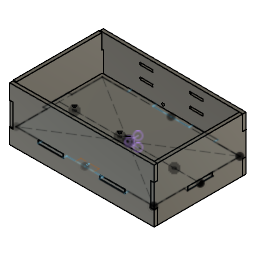
Backing Plate and Box (Autodesk Fusion 360 design; units mm, degrees)
part number: 2026-02-17-21-20-32-268
Autodesk Fusion 360 part; units mm, degrees
sketch "Base Plate" plane through (0, 0, 0) normal (0, 0, 1) x (1, 0, 0)
  line L0 (136.5, 85.5) -> (-136.5, 85.5) construction
  line L1 (-136.5, 85.5) -> (-136.5, -85.5) construction
  line L2 (-136.5, -85.5) -> (136.5, -85.5) construction
  line L3 (136.5, -85.5) -> (136.5, 85.5) construction
  line L4 (136.5, 85.5) -> (-136.5, -85.5) construction
  line L5 (-136.5, 85.5) -> (136.5, -85.5) construction
  line L6 (-35.8624, -85.7255) -> (-35.8624, -92.1)
  line L7 (-35.8624, -92.1) -> (-85.8619, -92.1)
  line L8 (-85.8619, -92.1) -> (-85.8619, -85.5)
  line L9 (-136.5, -85.5) -> (-85.8619, -85.5)
  line L10 (-35.8624, -85.7255) -> (0, -85.5)
  line L11 (0, 2.5) -> (0, 20)
  line L12 (136.5, -85.5) -> (85.8619, -85.5)
  line L13 (85.8619, -92.1) -> (85.8619, -85.5)
  line L14 (35.8624, -92.1) -> (85.8619, -92.1)
  line L15 (35.8624, -85.7255) -> (35.8624, -92.1)
  line L16 (35.8624, -85.7255) -> (0, -85.5)
  line L17 (20, 0) -> (2.5, 0)
  line L18 (-35.8624, 85.7255) -> (-35.8624, 92.1)
  line L19 (35.8624, 85.7255) -> (0, 85.5)
  line L20 (-136.5, 85.5) -> (136.5, 85.5) construction
  line L21 (-35.8624, 92.1) -> (-85.8619, 92.1)
  line L22 (35.8624, 92.1) -> (85.8619, 92.1)
  line L23 (136.5, 85.5) -> (85.8619, 85.5)
  line L24 (-136.5, 85.5) -> (-85.8619, 85.5)
  line L25 (35.8624, 85.7255) -> (35.8624, 92.1)
  line L26 (-35.8624, 85.7255) -> (0, 85.5)
  line L27 (-85.8619, 92.1) -> (-85.8619, 85.5)
  line L28 (85.8619, 92.1) -> (85.8619, 85.5)
  line L29 (-136.5, 25) -> (-143.1, 25)
  line L30 (-143.1, 25) -> (-143.1, 0)
  line L31 (-136.5, 25) -> (-136.5, 85.5)
  line L32 (-136.5, -25) -> (-136.5, -85.5)
  line L33 (-143.1, -25) -> (-143.1, 0)
  line L34 (-136.5, -25) -> (-143.1, -25)
  line L35 (136.5, -25) -> (143.1, -25)
  line L36 (143.1, -25) -> (143.1, 0)
  line L37 (136.5, 25) -> (136.5, 85.5)
  line L38 (136.5, -25) -> (136.5, -85.5)
  line L39 (143.1, 25) -> (143.1, 0)
  line L40 (136.5, 85.5) -> (136.5, -85.5) construction
  line L41 (136.5, 25) -> (143.1, 25)
  line L42 (-136.5, -85.5) -> (-136.5, 0.3) construction
  line L43 (-136.5, 0.3) -> (136.5, 0.3) construction
  line L44 (-136.5, 0.3) -> (-106.5, 0.3) construction
  line L45 (-106.5, 0.3) -> (-16.5, 0.3) construction
  line L46 (-16.5, 0.3) -> (91.5, 0.3) construction
  line L47 (91.5, 0.3) -> (136.5, 0.3) construction
  circle A0 centre (-106.5, 0.3) radius 2.45
  circle A1 centre (-16.5, 0.3) radius 2.45
  circle A2 centre (91.5, 0.3) radius 2.45
  line L48 (-17.9312, -85.6127) -> (17.9312, -85.6127) construction
  line L49 (17.9312, -85.6127) -> (17.9312, -75.542) construction
  line L50 (17.9312, -75.542) -> (-17.9312, -75.542) construction
  line L51 (-17.9312, -75.542) -> (-17.9312, -85.6127) construction
  point P0 (-136.5, -85.5)
  point P1 (136.5, -85.5)
  dimension "d1" = 273
  dimension "d2" = 171
  dimension "d3" = 50
  dimension "d4" = 6.6
  dimension "d6" = 6.6
  dimension "d7" = 25
  dimension "d8" = 85.8
  dimension "d9" = 273
  dimension "d10" = 30
  dimension "d11" = 90
  dimension "d12" = 108
  dimension "d13" = 45
  dimension "d16" = 4.9
  dimension "d17" = 4.9
  dimension "d18" = 4.9
  dimension "d23" = 7
  text T0 "B" font "Arial" height 7 align centre top in box 35.8624 x 10.0707 at (-17.9312, -85.6127) x (1, 0) y (0, 1) spacing 1 kerned
  constraint horizontal L0
  constraint perpendicular L0 L1
  constraint parallel L0 L2
  constraint parallel L1 L3
  constraint coincident L4 origin
  constraint coincident L5 origin
  constraint vertical L6
  constraint horizontal L7
  constraint vertical L8
  constraint coincident L2 L8.end
  constraint midpoint L2 L10.end
  constraint symmetric P0 L11 P1
  constraint symmetric L8.end L11 L12.end
  constraint symmetric L6.start L11 L15.start
  constraint symmetric L6.end L11 L14.start
  constraint symmetric L7.end L11 L13.start
  constraint symmetric L10.end L11 L16.end
  constraint symmetric P0 L17 L0.end
  constraint symmetric P1 L17 L0.start
  constraint symmetric L8.end L17 L24.end
  constraint symmetric L6.start L17 L18.start
  constraint symmetric L6.end L17 L18.end
  constraint symmetric L7.end L17 L21.end
  constraint symmetric L10.end L17 L19.end
  constraint symmetric L12.end L17 L23.end
  constraint symmetric L13.start L17 L22.end
  constraint symmetric L14.start L17 L22.start
  constraint symmetric L15.start L17 L19.start
  constraint perpendicular L29 L30
  constraint symmetric L0.end L17 P0
  constraint symmetric L17 L0.end P0
  constraint symmetric L17 L29.start L32.start
  constraint symmetric L17 L29.end L33.start
  constraint symmetric L17 L30.end L33.end
  constraint symmetric L0.end L11 L0.start
  constraint symmetric L11 L0.end L0.start
  constraint symmetric L11 L29.start L37.start
  constraint symmetric L11 L29.end L39.start
  constraint symmetric L11 L30.end L36.end
  constraint symmetric L11 P0 P1
  constraint symmetric L11 L32.start L35.start
  constraint symmetric L11 L33.start L35.end
  constraint parallel L1 L42
  constraint horizontal L43
  constraint horizontal L44
  constraint perpendicular L1 L45
  constraint horizontal L46
  constraint perpendicular L29 L31
  constraint coincident L30.end L33.end
  constraint perpendicular L0 L31
  constraint coincident L44.end L45.start
  constraint coincident L45.end L46.start
  constraint coincident L46.end L47.start
  constraint midpoint L16
  constraint midpoint L10
  measures "d1" distance of P0 P1
  measures "d2" distance of L0.end P0
  measures "d3" distance of L8.end L6.start
  measures "d4" distance of L8.end L7.end
  measures "d6" distance of L29.start L29.end
  measures "d7" distance of L29.end L30.end
  measures "d8" distance of P0 L42.end
  measures "d9" distance of L42.end L43.end
  measures "d10" distance of L42.end L44.end
  measures "d11" distance of L44.end L45.end
  measures "d12" distance of L45.end L46.end
  measures "d13" distance of L43.end L46.end
  measures "d16" diameter of A0
  measures "d17" diameter of A1
  measures "d18" diameter of A2
extrude "Extrude1" add sketch "Base Plate" along normal blind 6.6 makes body 1
fillet "Fillet1" radius 1 16 edges at (-85.8619, -92.1, 3.3) (-35.8624, -92.1, 3.3) (35.8624, -92.1, 3.3) (85.8619, -92.1, 3.3) (136.5, -85.5, 3.3) (-136.5, -85.5, 3.3) (-143.1, -25, 3.3) (-143.1, 25, 3.3) (-136.5, 85.5, 3.3) (-85.8619, 92.1, 3.3) (-35.8624, 92.1, 3.3) (35.8624, 92.1, 3.3) (85.8619, 92.1, 3.3) (136.5, 85.5, 3.3) (143.1, 25, 3.3) (143.1, -25, 3.3) on bodies 1
extrude "Extrude2" cut sketch "Base Plate" along normal blind 6.6 text T0 bodies 1 makes body 2 at (-1.7166, -77.0732, 2.2) makes body 3 at (36.9029, -29.1248, 0)
sketch "For Cutting" plane through (0, 0, 6.6) normal (0, 0, 1) x (-1, 0, 0)
  line L0 (2.6429, 82.542) -> (2.6429, 75.542)
  line L1 (2.6429, 75.542) -> (0.0167, 75.542)
  spline S0 degree 3 poles (0.0167, 75.542) (-0.2266, 75.5465) (-0.6666, 75.5545) (-1.0836, 75.6927) (-1.2701, 75.7545) knots 0 0 0 0 0.072475 0.131086 0.131086 0.131086 0.131086
  spline S1 degree 3 poles (-1.2701, 75.7545) (-1.4227, 75.8345) (-1.7265, 75.9939) (-1.9287, 76.2708) (-2.0293, 76.4087) knots 0 0 0 0 0.050943 0.101413 0.101413 0.101413 0.101413
  spline S2 degree 3 poles (-2.0293, 76.4087) (-2.1094, 76.5559) (-2.2664, 76.8446) (-2.2916, 77.1721) (-2.3039, 77.3326) knots 0 0 0 0 0.049654 0.097362 0.097362 0.097362 0.097362
  spline S3 degree 3 poles (-2.3039, 77.3326) (-2.2934, 77.4806) (-2.2721, 77.7795) (-2.1314, 78.0442) (-2.0604, 78.1778) knots 0 0 0 0 0.043994 0.088828 0.088828 0.088828 0.088828
  spline S4 degree 3 poles (-2.0604, 78.1778) (-1.9655, 78.3051) (-1.7672, 78.5714) (-1.4766, 78.7332) (-1.325, 78.8176) knots 0 0 0 0 0.047078 0.098463 0.098463 0.098463 0.098463
  spline S5 degree 3 poles (-1.325, 78.8176) (-1.5218, 78.8871) (-1.899, 79.0205) (-2.1712, 79.3128) (-2.3015, 79.4527) knots 0 0 0 0 0.061554 0.118026 0.118026 0.118026 0.118026
  spline S6 degree 3 poles (-2.3015, 79.4527) (-2.4011, 79.6112) (-2.6046, 79.9352) (-2.63, 80.3174) (-2.6429, 80.5127) knots 0 0 0 0 0.055236 0.112931 0.112931 0.112931 0.112931
  spline S7 degree 3 poles (-2.6429, 80.5127) (-2.6346, 80.6729) (-2.6183, 80.9898) (-2.4958, 81.2824) (-2.4352, 81.4271) knots 0 0 0 0 0.047734 0.094399 0.094399 0.094399 0.094399
  spline S8 degree 3 poles (-2.4352, 81.4271) (-2.3649, 81.5575) (-2.2317, 81.805) (-2.0213, 81.9909) (-1.9219, 82.0789) knots 0 0 0 0 0.044041 0.083545 0.083545 0.083545 0.083545
  spline S9 degree 3 poles (-1.9219, 82.0789) (-1.8097, 82.1515) (-1.5719, 82.3055) (-1.2994, 82.3837) (-1.1555, 82.425) knots 0 0 0 0 0.039883 0.084504 0.084504 0.084504 0.084504
  spline S10 degree 3 poles (-1.1555, 82.425) (-0.9851, 82.4591) (-0.6126, 82.5336) (-0.2325, 82.539) (-0.0263, 82.542) knots 0 0 0 0 0.052016 0.113741 0.113741 0.113741 0.113741
  line L2 (-0.0263, 82.542) -> (2.6429, 82.542)
  arc A0 (-142.1, 25) -> (-143.1, 24) centre (-142.1, 24) ccw
  line L3 (-143.1, 24) -> (-143.1, -24)
  arc A1 (-143.1, -24) -> (-142.1, -25) centre (-142.1, -24) ccw
  line L4 (-142.1, -25) -> (-136.5, -25)
  line L5 (-136.5, -25) -> (-136.5, -84.5)
  arc A2 (-136.5, -84.5) -> (-135.5, -85.5) centre (-135.5, -84.5) ccw
  line L6 (-135.5, -85.5) -> (-85.8619, -85.5)
  line L7 (-85.8619, -85.5) -> (-85.8619, -91.1)
  arc A3 (-85.8619, -91.1) -> (-84.8619, -92.1) centre (-84.8619, -91.1) ccw
  line L8 (-84.8619, -92.1) -> (-36.8624, -92.1)
  arc A4 (-36.8624, -92.1) -> (-35.8624, -91.1) centre (-36.8624, -91.1) ccw
  line L9 (-35.8624, -91.1) -> (-35.8624, -85.7255)
  line L10 (-35.8624, -85.7255) -> (0, -85.5)
  line L11 (0, -85.5) -> (35.8624, -85.7255)
  line L12 (35.8624, -85.7255) -> (35.8624, -91.1)
  arc A5 (35.8624, -91.1) -> (36.8624, -92.1) centre (36.8624, -91.1) ccw
  line L13 (36.8624, -92.1) -> (84.8619, -92.1)
  arc A6 (84.8619, -92.1) -> (85.8619, -91.1) centre (84.8619, -91.1) ccw
  line L14 (85.8619, -91.1) -> (85.8619, -85.5)
  line L15 (85.8619, -85.5) -> (135.5, -85.5)
  arc A7 (135.5, -85.5) -> (136.5, -84.5) centre (135.5, -84.5) ccw
  line L16 (136.5, -84.5) -> (136.5, -25)
  line L17 (136.5, -25) -> (142.1, -25)
  arc A8 (142.1, -25) -> (143.1, -24) centre (142.1, -24) ccw
  line L18 (143.1, -24) -> (143.1, 24)
  arc A9 (143.1, 24) -> (142.1, 25) centre (142.1, 24) ccw
  line L19 (142.1, 25) -> (136.5, 25)
  line L20 (136.5, 25) -> (136.5, 84.5)
  arc A10 (136.5, 84.5) -> (135.5, 85.5) centre (135.5, 84.5) ccw
  line L21 (135.5, 85.5) -> (85.8619, 85.5)
  line L22 (85.8619, 85.5) -> (85.8619, 91.1)
  arc A11 (85.8619, 91.1) -> (84.8619, 92.1) centre (84.8619, 91.1) ccw
  line L23 (84.8619, 92.1) -> (36.8624, 92.1)
  arc A12 (36.8624, 92.1) -> (35.8624, 91.1) centre (36.8624, 91.1) ccw
  line L24 (35.8624, 91.1) -> (35.8624, 85.7255)
  line L25 (35.8624, 85.7255) -> (0, 85.5)
  line L26 (0, 85.5) -> (-35.8624, 85.7255)
  line L27 (-35.8624, 85.7255) -> (-35.8624, 91.1)
  arc A13 (-35.8624, 91.1) -> (-36.8624, 92.1) centre (-36.8624, 91.1) ccw
  line L28 (-36.8624, 92.1) -> (-84.8619, 92.1)
  arc A14 (-84.8619, 92.1) -> (-85.8619, 91.1) centre (-84.8619, 91.1) ccw
  line L29 (-85.8619, 91.1) -> (-85.8619, 85.5)
  line L30 (-85.8619, 85.5) -> (-135.5, 85.5)
  arc A15 (-135.5, 85.5) -> (-136.5, 84.5) centre (-135.5, 84.5) ccw
  line L31 (-136.5, 84.5) -> (-136.5, 25)
  line L32 (-136.5, 25) -> (-142.1, 25)
  circle A16 centre (106.5, -0.3) radius 2.45
  circle A17 centre (16.5, -0.3) radius 2.45
  circle A18 centre (-91.5, -0.3) radius 2.45
sketch "Top/Bottom Plate" plane through (0.5375, 85.4966, 0) normal (0.006286, 0.99998, 0) x (-0.99998, 0.006286, 0)
  line L0 (36.4006, 0) -> (36.4006, 6.6)
  line L1 (36.4344, 6.6) -> (36.4344, 0)
  line L2 (86.4329, 0) -> (86.4329, 6.6)
  line L3 (-85.2875, 6.6) -> (-85.2875, 0)
  line L4 (-35.289, 0) -> (-35.289, 6.6)
  line L5 (37.4407, 6.6) -> (85.4392, 6.6)
  line L6 (36.4407, 0) -> (86.4392, 0)
  line L7 (-35.2827, 0) -> (-85.2812, 0)
  line L8 (-84.2813, 6.6) -> (-36.2827, 6.6)
  line L9 (-135.9661, 6.6) -> (-135.9661, 0)
  line L10 (137.0285, 0) -> (137.0285, 6.6)
  line L11 (-85.2875, 6.6) -> (-35.289, 6.6)
  line L12 (-35.289, 6.6) -> (-35.289, 0)
  line L13 (-35.289, 0) -> (-85.2875, 0)
  line L14 (-85.2875, 0) -> (-85.2875, 6.6)
  line L15 (36.4344, 6.6) -> (86.4329, 6.6)
  line L16 (86.4329, 6.6) -> (86.4329, 0)
  line L17 (86.4329, 0) -> (36.4344, 0)
  line L18 (-135.9661, 6.6) -> (-135.9661, 76.6) construction
  line L19 (-135.9661, 0) -> (-135.9661, -30) construction
  line L20 (137.0285, 6.6) -> (137.0285, 76.6) construction
  line L21 (137.0285, 0) -> (137.0285, -30) construction
  line L22 (-135.9661, 76.6) -> (137.0285, 76.6)
  line L23 (137.0285, 76.6) -> (137.0285, -30) construction
  line L24 (137.0285, -30) -> (-135.9661, -30)
  line L25 (-135.9661, -30) -> (-135.9661, 76.6) construction
  line L26 (-135.9661, 76.6) -> (-142.5661, 76.6)
  line L27 (-142.5661, 76.6) -> (-142.5661, 46.6)
  line L28 (-142.5661, 46.6) -> (-135.9661, 46.6)
  line L29 (-135.9661, -30) -> (-142.5661, -30)
  line L30 (-142.5661, -30) -> (-142.5661, 0)
  line L31 (-142.5661, 0) -> (-135.9661, 0)
  line L32 (-135.9661, 0) -> (-135.9661, 46.6)
  line L33 (0, 1.75) -> (0, 22.5)
  line L34 (135.9661, 76.6) -> (142.5661, 76.6)
  line L35 (142.5661, 76.6) -> (142.5661, 46.6)
  line L36 (142.5661, 46.6) -> (135.9661, 46.6)
  line L37 (135.9661, 0) -> (135.9661, 46.6)
  line L38 (142.5661, 0) -> (135.9661, 0)
  line L39 (142.5661, -30) -> (142.5661, 0)
  line L40 (135.9661, -30) -> (142.5661, -30)
  dimension "d27" = 70
  dimension "d28" = 30
  dimension "d29" = 70
  dimension "d30" = 30
  dimension "d33" = 6.6
  dimension "d34" = 30
  dimension "d35" = 6.6
  dimension "d36" = 30
  constraint horizontal L11
  constraint vertical L12
  constraint horizontal L13
  constraint vertical L14
  constraint coincident L4.start L12.end
  constraint coincident L3.start L11.start
  constraint horizontal L15
  constraint vertical L16
  constraint horizontal L17
  constraint coincident L2.start L16.end
  constraint coincident L1.start L15.start
  constraint vertical L18
  constraint coincident L9.start L18.start
  constraint coincident L9.end L19.start
  constraint parallel L9 L19
  constraint coincident L10.end L20.start
  constraint parallel L10 L20
  constraint coincident L10.start L21.start
  constraint parallel L10 L21
  constraint horizontal L22
  constraint vertical L23
  constraint horizontal L24
  constraint vertical L25
  constraint horizontal L26
  constraint vertical L27
  constraint horizontal L28
  constraint horizontal L29
  constraint vertical L30
  constraint horizontal L31
  constraint symmetric L18.end L33 L34.start
  constraint symmetric L9.end L33 L37.start
  constraint symmetric L19.end L33 L40.start
  constraint symmetric L26.end L33 L34.end
  constraint symmetric L27.end L33 L35.end
  constraint symmetric L28.end L33 L36.end
  constraint symmetric L29.end L33 L39.start
  constraint symmetric L30.end L33 L38.start
  measures "d27" distance of L9.start L18.end
  measures "d28" distance of L9.end L19.end
  measures "d29" distance of L10.end L20.end
  measures "d30" distance of L10.start L21.end
  measures "d33" distance of L18.end L26.end
  measures "d34" distance of L18.end L28.end
  measures "d35" distance of L19.end L29.end
  measures "d36" distance of L19.end L9.end
extrude "Extrude5" add sketch "Top/Bottom Plate" along normal blind 6.6 separate body makes body 4
mirror "Mirror2" about plane through (0, 0, 0) normal (0, 1, 0) of bodies 4 makes body 5
sketch "Left/Right Plate" plane through (136.5, 0, 0) normal (1, 0, 0) x (0, 1, 0)
  line L0 (25, 0) -> (25, 6.6)
  line L1 (-25, 6.6) -> (-25, 0)
  line L2 (-84.6004, 0) -> (-91.2002, 0)
  line L3 (-84.6004, 46.6) -> (-91.2002, 46.6)
  line L4 (84.6004, 46.6) -> (91.2002, 46.6)
  line L5 (84.6004, 0) -> (91.2002, 0)
  line L6 (-84.6004, 76.6) -> (84.6004, 76.6)
  line L7 (84.6004, 76.6) -> (84.6004, -30) construction
  line L8 (84.6004, -30) -> (-84.6004, -30)
  line L9 (-84.6004, -30) -> (-84.6004, 76.6) construction
  line L10 (-91.2002, 46.6) -> (-84.6004, 46.6)
  line L11 (-84.6004, 0) -> (-91.2002, 0)
  line L12 (-91.2002, 0) -> (-91.2002, 46.6)
  line L13 (84.6004, 46.6) -> (91.2002, 46.6)
  line L14 (91.2002, 46.6) -> (91.2002, 0)
  line L15 (91.2002, 0) -> (84.6004, 0)
  line L16 (-84.6004, 46.6) -> (-84.6004, 76.6)
  line L17 (-84.6004, 0) -> (-84.6004, -30)
  line L18 (84.6004, 0) -> (84.6004, -30)
  line L19 (84.6004, 46.6) -> (84.6004, 76.6)
  line L20 (-25, 6.6) -> (25, 6.6)
  line L21 (25, 6.6) -> (25, 0)
  line L22 (25, 0) -> (-25, 0)
  line L23 (-25, 0) -> (-25, 6.6)
  point P0 (-84.6004, 76.6)
  point P1 (-84.6004, -30)
  point P2 (84.6004, -30)
  point P3 (84.6004, 76.6)
  point P4 (-84.6004, 46.6)
  point P5 (-91.2002, 0)
  point P6 (91.2002, 0)
  point P7 (84.6419, 46.6)
  constraint horizontal L6
  constraint vertical L7
  constraint horizontal L8
  constraint vertical L9
  constraint coincident P2 L7.end
  constraint coincident P0 L6.start
  constraint horizontal L10
  constraint horizontal L11
  constraint vertical L12
  constraint coincident L2.start L11.start
  constraint coincident L3.end L10.start
  constraint horizontal L13
  constraint vertical L14
  constraint horizontal L15
  constraint coincident P6 L5.end
  constraint coincident L4.start L13.start
  constraint coincident P4 L3.start
  constraint coincident P1 L8.end
  constraint coincident L5.start L15.end
  constraint coincident P3 L6.end
  constraint horizontal L20
  constraint vertical L21
  constraint horizontal L22
  constraint vertical L23
  constraint coincident L0.start L21.end
  constraint coincident L1.start L20.start
extrude "Extrude6" add sketch "Left/Right Plate" along normal blind 6.6 separate body makes body 6
mirror "Mirror3" about plane through (0, 0, 0) normal (1, 0, 0) of bodies 6 makes body 7
sketch "Top Plate Detail" plane through (0.579, 92.0965, 0) normal (0.006286, 0.99998, 0) x (-0.99998, 0.006286, 0)
  line L0 (36.4344, 0) -> (36.4344, 6.6)
  line L1 (36.4344, 6.6) -> (86.4329, 6.6)
  line L2 (86.4329, 6.6) -> (86.4329, 0)
  line L3 (86.4329, 0) -> (36.4344, 0)
  line L4 (-35.289, 0) -> (-85.2875, 0)
  line L5 (-85.2875, 0) -> (-85.2875, 6.6)
  line L6 (-85.2875, 6.6) -> (-35.289, 6.6)
  line L7 (-35.289, 6.6) -> (-35.289, 0)
  line L8 (-142.5661, -30) -> (142.5661, -30)
  line L9 (142.5661, -30) -> (142.5661, 0)
  line L10 (142.5661, 0) -> (135.9661, 0)
  line L11 (135.9661, 0) -> (135.9661, 46.6)
  line L12 (135.9661, 46.6) -> (142.5661, 46.6)
  line L13 (142.5661, 46.6) -> (142.5661, 76.6)
  line L14 (142.5661, 76.6) -> (-142.5661, 76.6)
  line L15 (-142.5661, 76.6) -> (-142.5661, 46.6)
  line L16 (-142.5661, 46.6) -> (-135.9661, 46.6)
  line L17 (-135.9661, 46.6) -> (-135.9661, 0)
  line L18 (-135.9661, 0) -> (-142.5661, 0)
  line L19 (-142.5661, 0) -> (-142.5661, -30)
  line L20 (0, -30) -> (0, 76.6) construction
  line L21 (-91.4963, 0) -> (-91.4963, 13) construction
  line L22 (16.5016, 0) -> (16.5016, 13) construction
  circle A0 centre (-91.4963, 13) radius 2.6
  circle A1 centre (16.5016, 13) radius 2.6
  line L23 (0, 0) -> (-50, 0) construction
  line L24 (-50, 0) -> (-50, -15) construction
  line L25 (-37, -12.9) -> (-63, -12.9)
  line L26 (-63, -12.9) -> (-63, -17.1)
  line L27 (-63, -17.1) -> (-37, -17.1)
  line L28 (-37, -17.1) -> (-37, -12.9)
  line L29 (-37, -12.9) -> (-63, -17.1) construction
  line L30 (-63, -12.9) -> (-37, -17.1) construction
  line L31 (37, -12.9) -> (63, -12.9)
  line L32 (37, -17.1) -> (37, -12.9)
  line L33 (63, -17.1) -> (37, -17.1)
  line L34 (63, -12.9) -> (63, -17.1)
  line L35 (-37, 37.1) -> (-63, 37.1)
  line L36 (-37, 32.9) -> (-37, 37.1)
  line L37 (-63, 32.9) -> (-37, 32.9)
  line L38 (-63, 37.1) -> (-63, 32.9)
  line L39 (37, 32.9) -> (37, 37.1)
  line L40 (37, 37.1) -> (63, 37.1)
  line L41 (63, 32.9) -> (37, 32.9)
  line L42 (63, 37.1) -> (63, 32.9)
  line L43 (-63, 62.1) -> (-63, 57.9)
  line L44 (-63, 57.9) -> (-37, 57.9)
  line L45 (-37, 62.1) -> (-63, 62.1)
  line L46 (-37, 57.9) -> (-37, 62.1)
  line L47 (37, 57.9) -> (37, 62.1)
  line L48 (37, 62.1) -> (63, 62.1)
  line L49 (63, 57.9) -> (37, 57.9)
  line L50 (63, 62.1) -> (63, 57.9)
  point P0 (-91.4963, 0)
  point P1 (16.5016, 0)
  point P2 (-50, -15)
  dimension "d49" = 13
  dimension "d50" = 13
  dimension "d54" = 5.2
  dimension "d55" = 5.2
  dimension "d56" = 50
  dimension "d57" = 15
  dimension "d58" = 26
  dimension "d59" = 4.2
  dimension "d62" = 0
  dimension "d63" = 50
  dimension "d66" = 0
  dimension "d67" = 25
  constraint vertical L20
  constraint midpoint L8 L20.start
  constraint coincident L14 L20.end
  constraint vertical L21
  constraint coincident P0 L21.start
  constraint vertical L22
  constraint coincident P1 L22.start
  constraint coincident L21.end A0.centre
  constraint coincident L22.end A1.centre
  constraint coincident L23.start origin
  constraint perpendicular L7 L23
  constraint perpendicular L23 L24
  constraint horizontal L25
  constraint perpendicular L25 L26
  constraint parallel L25 L27
  constraint parallel L26 L28
  constraint coincident L29 P2
  constraint coincident L30 P2
  constraint coincident P2 L24.end
  constraint symmetric L20 L25.start L31.start
  constraint symmetric L20 L25.end L31.end
  constraint symmetric L20 L26.end L33.start
  constraint symmetric L20 L27.end L32.start
  measures "d49" distance of P0 L21.end
  measures "d50" distance of P1 L22.end
  measures "d54" diameter of A0
  measures "d55" diameter of A1
  measures "d56" distance of L23.start L23.end
  measures "d57" distance of L23.end P2
  measures "d58" distance of L26.end L27.end
  measures "d59" distance of L25.end L26.end
extrude "Extrude7" cut sketch "Top Plate Detail" against normal blind 6.6 contours A0 | A1 | L25 L26 L27 L28 | L31 L32 L33 L34 | L35 L36 L37 L38 | L39 L40 L41 L42 | L43 L44 L45 L46 | L47 L48 L49 L50 bodies 4
equation "d4 = thickness"
equation "d6 = thickness"
equation "thickness = 6.6 mm"
equation "dowel_hole_diameter = 4.9 mm"
equation "d16 = dowel_hole_diameter"
equation "d17 = dowel_hole_diameter"
equation "d18 = dowel_hole_diameter"
equation "d19 = thickness"
equation "d24 = 'B'"
equation "d25 = thickness"
equation "d33 = thickness"
equation "d35 = thickness"
equation "d39 = thickness"
equation "d45 = thickness"
equation "d49 = top_hole_distance"
equation "d50 = top_hole_distance"
equation "thickness_waves = 4.2 mm"
equation "duck_dowel_hole_diameter = 5.2 mm"
equation "top_hole_distance = 13 mm"
equation "d54 = duck_dowel_hole_diameter"
equation "d55 = duck_dowel_hole_diameter"
equation "d68 = -thickness"
named bodies: "B part", "B part (1)", "Base Plate", "Top Plate", "Bottom Plate", "Side Plate 1", "Side Plate 2"
